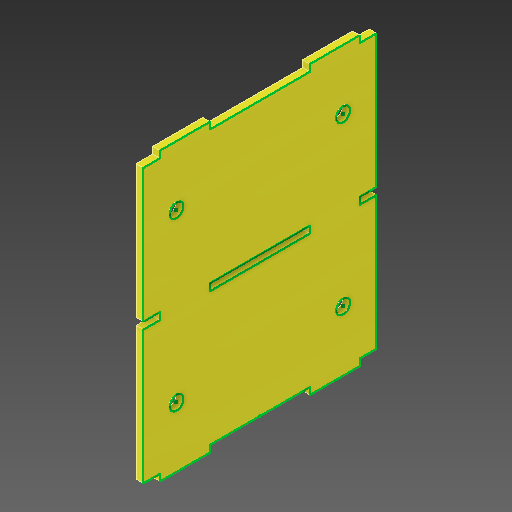
# Autodesk Inventor part: CH_01_0010_syringe_pump_servo
Saved by Autodesk Inventor 2022 (Build 260153000, 153)
## iProperties
Created: 2022-02-25
Part Number: CH_01_0010_syringe_pump_servo
Material: Aluminum 6061
Document SubType Name: Modeling
Designer: Tomasz Krakowski
Density: 2.7 g/cm^3
Appearance: Kanarkowa
Mass: 30.8685 g
Surface Area: 123.539 cm^2
Volume: 11.4328 cm^3
Author: Tomasz Krakowski
Autodesk Inventor part; units mm, degrees
ref_plane "YZ Plane" through (0, 0, 0) normal (1, 0, 0) x (0, 1, 0)
ref_plane "XZ Plane" through (0, 0, 0) normal (0, 1, 0) x (-1, 0, 0)
ref_plane "XY Plane" through (0, 0, 0) normal (0, 0, 1) x (1, 0, 0)
sketch "Sketch1" plane through (0, 0, 0) normal (1, 0, 0) x (0, 1, 0)
  line L0 (0, 15) -> (0, 0)
  line L1 (0, 15) -> (-2, 15)
  line L2 (-2, 15) -> (-2, 30)
  line L3 (-2, 30) -> (0, 30)
  line L4 (0, 30) -> (0, 35)
  line L5 (0, 35) -> (39.95, 35)
  line L6 (20, 0) -> (0, 0) construction
  line L7 (39.95, 35) -> (39.95, 30)
  line L8 (39.95, 30) -> (42.05, 30)
  line L9 (42.05, 15) -> (39.95, 15)
  line L10 (39.95, 15) -> (39.95, 0)
  line L11 (39.95, 0) -> (20, 0) construction
  line L12 (0, -15) -> (0, 0)
  line L13 (0, -15) -> (-2, -15)
  line L14 (-2, -15) -> (-2, -30)
  line L15 (-2, -30) -> (0, -30)
  line L16 (0, -30) -> (0, -35)
  line L17 (0, -35) -> (39.95, -35)
  line L18 (39.95, -35) -> (39.95, -30)
  line L19 (39.95, -30) -> (42.05, -30)
  line L20 (42.05, -15) -> (39.95, -15)
  line L21 (39.95, -15) -> (39.95, 0)
  line L22 (41, 30) -> (41, -30) construction
  line L23 (82, 15) -> (82, 0)
  line L24 (82, 15) -> (84, 15)
  line L25 (84, 30) -> (82, 30)
  line L26 (82, 30) -> (82, 35)
  line L27 (82, 35) -> (42.05, 35)
  line L28 (42.05, 35) -> (42.05, 30)
  line L29 (42.05, 15) -> (42.05, 0)
  line L30 (42.05, -35) -> (42.05, -30)
  line L31 (42.05, -15) -> (42.05, 0)
  line L32 (82, -15) -> (84, -15)
  line L33 (84, -15) -> (84, -30)
  line L34 (84, -30) -> (82, -30)
  line L35 (82, -30) -> (82, -35)
  line L36 (82, -15) -> (82, 0)
  line L37 (82, -35) -> (42.05, -35)
  line L38 (84, 30) -> (84, 15)
  dimension "d3" = 15
  dimension "d6" = 20
  dimension "d7" = 35
  dimension "d8" = 15
  dimension "d9" = 2
  dimension "d17" = 2.1
  dimension "d23" = 41
  constraints: 78 end point, 24 symmetric about line, 8 point on line, 5 perpendicular, 3 collinear, 3 horizontal, 3 vertical, 2 midpoint
  measures "d3" distance between parallel lines of L1 L3
  measures "d6" distance from line of L6.start L0
  measures "d7" distance between parallel lines of L6 L5
  measures "d8" distance between parallel lines of L6 L1
  measures "d9" distance between parallel lines of L0 L2
  measures "d17" distance between parallel lines of L7 L28
  measures "d23" distance between parallel lines of L22 L4
extrude "Wyciągnięcie proste1" add sketch "Sketch1" along normal blind 2
sketch "Szkic3" plane through (2, 0, 0) normal (1, 0, 0) x (0, 0, -1)
  line L0 (-25, 16) -> (25, 16) construction
  line L1 (25, 16) -> (25, 66) construction
  line L2 (25, 66) -> (-25, 66) construction
  line L3 (-25, 66) -> (-25, 16) construction
  line L4 (-25, 16) -> (25, 66) construction
  line L5 (25, 16) -> (-25, 66) construction
  line L6 (0, 41) -> (0, 42.05) construction
  line L7 (-15, 42.05) -> (15, 42.05) construction
  line L8 (0, 41) -> (15, 41) construction
  line L9 (15, 42.05) -> (15, 39.95) construction
  circle A0 centre (-25, 66) radius 2.1
  circle A1 centre (25, 66) radius 2.1
  circle A2 centre (25, 16) radius 2.1
  circle A3 centre (-25, 16) radius 2.1
  point P0 (0, 0)
  dimension "d18" = 4.2
  dimension "d19" = 50
  dimension "d20" = 50
  constraints: 16 end point, 4 centre point, 4 coincident, 4 midpoint, 3 equal radius, 3 perpendicular, 2 parallel, 1 horizontal
  measures "d18" diameter of A0
  measures "d19" distance of L1.end L2.end
  measures "d20" distance between parallel lines of L0 L2
extrude "Wyciągnięcie proste2" cut sketch "Szkic3" against normal up to surface (2 mm away)
sketch "Sketch4" plane through (2, 0, 0) normal (1, 0, 0) x (0, 0, -1)
  circle A0 centre (25, 16) radius 2.1 projected
  circle A1 centre (-25, 16) radius 2.1 projected
  circle A2 centre (25, 66) radius 2.1 projected
  circle A3 centre (-25, 66) radius 2.1 projected
  line L0 (-15, 42.05) -> (15, 42.05) projected
  line L1 (15, 42.05) -> (15, 39.95) projected
  line L2 (15, 39.95) -> (-15, 39.95) projected
  line L3 (-15, 39.95) -> (-15, 42.05) projected
  line L4 (-15, 0) -> (15, 0) projected
  line L5 (15, 0) -> (15, -2) projected
  line L6 (15, -2) -> (30, -2) projected
  line L7 (30, -2) -> (30, 0) projected
  line L8 (30, 0) -> (35, 0) projected
  line L9 (35, 0) -> (35, 39.95) projected
  line L10 (35, 39.95) -> (30, 39.95) projected
  line L11 (30, 39.95) -> (30, 42.05) projected
  line L12 (30, 42.05) -> (35, 42.05) projected
  line L13 (35, 42.05) -> (35, 82) projected
  line L14 (35, 82) -> (30, 82) projected
  line L15 (30, 82) -> (30, 84) projected
  line L16 (30, 84) -> (15, 84) projected
  line L17 (15, 84) -> (15, 82) projected
  line L18 (15, 82) -> (-15, 82) projected
  line L19 (-15, 82) -> (-15, 84) projected
  line L20 (-15, 84) -> (-30, 84) projected
  line L21 (-30, 84) -> (-30, 82) projected
  line L22 (-30, 82) -> (-35, 82) projected
  line L23 (-35, 82) -> (-35, 42.05) projected
  line L24 (-35, 42.05) -> (-30, 42.05) projected
  line L25 (-30, 42.05) -> (-30, 39.95) projected
  line L26 (-30, 39.95) -> (-35, 39.95) projected
  line L27 (-35, 39.95) -> (-35, 0) projected
  line L28 (-35, 0) -> (-30, 0) projected
  line L29 (-30, 0) -> (-30, -2) projected
  line L30 (-30, -2) -> (-15, -2) projected
  line L31 (-15, -2) -> (-15, 0) projected
  point P0 (0, 0)
equation "\"d6\" = 0.5 * d10"
equation "\"d10\" = 40"
